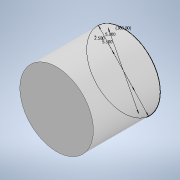
# Autodesk Inventor part: Powder Canister
Saved by Autodesk Inventor 2021 (Build 250183000, 183)
## iProperties
Created: 2021-01-08
Part Number: Powder Canister
Material: Generic
Document SubType Name: Modeling
Designer: saipr
Density: 1 g/cm^3
Appearance: Default
Author: saipr
Autodesk Inventor part; units mm, degrees
ref_plane "YZ Plane" through (0, 0, 0) normal (1, 0, 0) x (0, 1, 0)
ref_plane "XZ Plane" through (0, 0, 0) normal (0, 1, 0) x (-1, 0, 0)
ref_plane "XY Plane" through (0, 0, 0) normal (0, 0, 1) x (1, 0, 0)
sketch "Sketch1" plane through (0, 0, 0) normal (0, 0, 1) x (1, 0, 0)
  circle A0 centre (0, 0) radius 31.75
  circle A1 centre (0, 0) radius 63.5
  circle A2 centre (0, 0) radius 69.85
  line L0 (0, 0) -> (0, 69.85)
  line L1 (0, 0) -> (-60.4919, 34.925)
  line L2 (0, 0) -> (-60.4919, -34.925)
  line L3 (0, 0) -> (0, -69.85)
  line L4 (0, 0) -> (60.4919, -34.925)
  line L5 (0, 0) -> (60.4919, 34.925)
  point P0 (54.9926, 31.75)
  point P1 (27.4963, 15.875)
  point P2 (27.4963, -15.875)
  point P3 (54.9926, -31.75)
  point P4 (0, -63.5)
  point P5 (0, -31.75)
  point P6 (-27.4963, -15.875)
  point P7 (-54.9926, -31.75)
  point P8 (-54.9926, 31.75)
  point P9 (-27.4963, 15.875)
  point P10 (0, 31.75)
  point P11 (0, 63.5)
  dimension "d16" = 139.7
  dimension "d5" = 360
  dimension "d14" = 127
  dimension "d15" = 63.5
  constraints: 12 end point, 3 coincident, 2 centre point, 1 vertical, 1 vertical alignment, 21 other
  measures "d14" diameter of A1
  measures "d15" diameter of A0
extrude "Extrusion1" add sketch "Sketch1" along normal blind 127 contours L5 A2 L4 A1 | A1 L0 A2 L5 | L4 A2 L3 A1 | A1 L1 A2 L0 | L3 A2 L2 A1 | A1 L2 A2 L1
extrude "Extrusion2" add sketch "Sketch1" along normal blind 6.35 contours A0 L5 A1 L4 | A0 L1 A1 L0 | L3 A1 L2 A0
sketch "Sketch2" plane through (0, 0, 127) normal (0, 0, 1) x (1, 0, 0)
  arc A0 (54.9926, 31.75) -> (0, 63.5) centre (0, 0) ccw projected
  circle A1 centre (0, 0) radius 63.5
  point P0 (54.9926, 31.75)
  constraints: 1 coincident, 3 other
extrude "Extrusion3" add sketch "Sketch2" against normal blind 3.175
body "Solid1"
